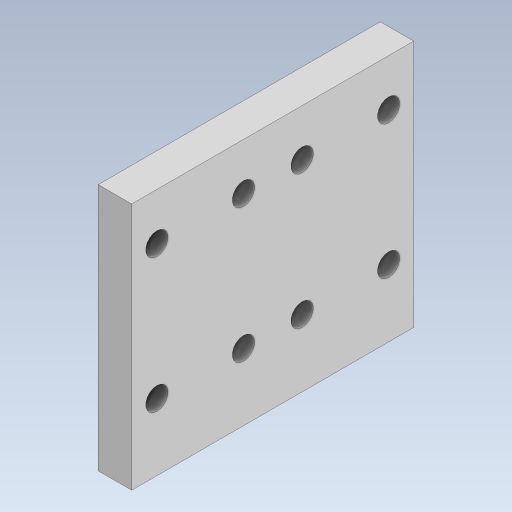
# Autodesk Inventor part: Konektor Lifter
Saved by Autodesk Inventor 2023.5 (Build 275446000, 446)
## iProperties
Created: 2025-09-06
Part Number: Konektor Lifter
Material: Generic
Document SubType Name: Modeling
Designer: Guntur
Density: 1 g/cm^3
Appearance: Default
Author: Guntur
Autodesk Inventor part; units mm, degrees
ref_plane "YZ Plane" through (0, 0, 0) normal (1, 0, 0) x (0, 1, 0)
ref_plane "XZ Plane" through (0, 0, 0) normal (0, 1, 0) x (-1, 0, 0)
ref_plane "XY Plane" through (0, 0, 0) normal (0, 0, 1) x (1, 0, 0)
sketch "Sketch1" plane through (0, 0, 0) normal (1, 0, 0) x (0, 1, 0)
  line L0 (11.1, 12.625) -> (-11.1, 12.625)
  line L1 (-11.1, 12.625) -> (-11.1, -12.625)
  line L2 (-11.1, -12.625) -> (11.1, -12.625)
  line L3 (11.1, -12.625) -> (11.1, 12.625)
  line L4 (7.1853, 0) -> (-6.35, 0) construction
  line L5 (0, 7.4808) -> (0, -6.6937) construction
  circle A0 centre (-5.1, 10.375) radius 1
  circle A1 centre (-5.1, 2.625) radius 1
  circle A2 centre (-5.1, -10.375) radius 1
  circle A3 centre (-5.1, -2.625) radius 1
  circle A4 centre (6.9, 10.375) radius 1
  circle A5 centre (6.9, -10.375) radius 1
  circle A6 centre (6.9, 2.625) radius 1
  circle A7 centre (6.9, -2.625) radius 1
  point P0 (0, 0)
  dimension "d0" = 22.2
  dimension "d1" = 25.25
  dimension "d2" = 2
  dimension "d3" = 6
  dimension "d4" = 2.25
  dimension "d5" = 2
  dimension "d6" = 10
  dimension "d9" = 2
  dimension "d10" = 4.2
  dimension "d14" = 2
  dimension "d15" = 2
  constraints: 12 end point, 8 centre point, 3 symmetric about line, 2 parallel, 1 horizontal, 1 perpendicular, 1 vertical, 3 other
  measures "d0" distance of L2.end L1.end
  measures "d1" distance of L1.end L0.end
  measures "d2" diameter of A0
  measures "d3" distance from line of L1 A0.centre
  measures "d4" distance from line of L0 A0.centre
  measures "d5" diameter of A1
  measures "d6" distance from line of L0 A1.centre
  measures "d9" diameter of A4
  measures "d10" distance from line of L3 A4.centre
  measures "d14" diameter of A6
  measures "d15" diameter of A7
extrude "Extrusion1" add sketch "Sketch1" along normal blind 3 contours L3 L2 L1 L0 | A6 | A7
extrude "Extrusion2" cut sketch "Sketch1" along normal blind 3 contours A6 | A7
body "Solid1"
